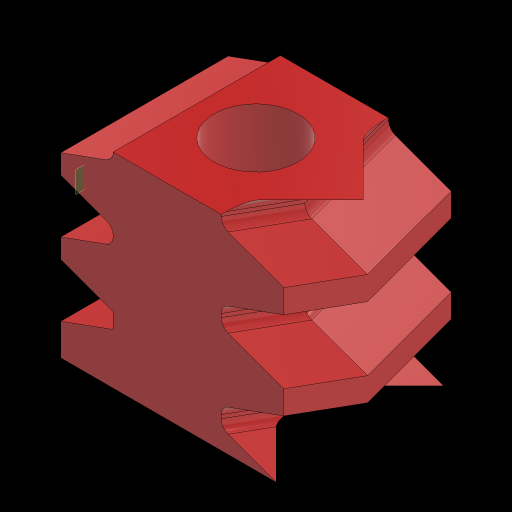
# Autodesk Inventor part: rack
Saved by Autodesk Inventor 2023.2 (Build 272271030, 271C)
## iProperties
Created: 2023-10-23
Part Number: rack
Material: Generic
Document SubType Name: Modeling
Designer: robpl
Density: 1 g/cm^3
Appearance: Red
Author: robpl
## iProperties of the stored document rack_3DPrint.ipt
Created: 2023-10-23
Part Number: rack_3DPrint
Material: Generic
Document SubType Name: Modeling
Designer: robpl
Density: 1 g/cm^3
Appearance: Default
Author: robpl
Autodesk Inventor part; units mm, degrees
ref_plane "YZ Plane" through (0, 0, 0) normal (1, 0, 0) x (0, 1, 0)
ref_plane "XZ Plane" through (0, 0, 0) normal (0, 1, 0) x (-1, 0, 0)
ref_plane "XY Plane" through (0, 0, 0) normal (0, 0, 1) x (1, 0, 0)
sketch "Sketch1" plane through (0, 0, 0) normal (0, 0, 1) x (1, 0, 0)
  line L0 (-6, -5.5) -> (6, -5.5)
  line L1 (6, -5.5) -> (6, 5.5)
  line L2 (6, 5.5) -> (-6, 5.5)
  line L3 (-6, 5.5) -> (-6, -5.5)
  point P0 (0, 0)
  point P1 (-6, 0)
  point P2 (0, 5.5)
  dimension "d0" = 12
  dimension "d1" = 11
  constraints: 8 end point, 2 midpoint, 2 parallel, 1 horizontal, 1 horizontal alignment, 1 perpendicular, 1 vertical alignment
  measures "d0" distance of L2.end L1.end
  measures "d1" distance of L1.end L0.end
extrude "Extrusion1" add sketch "Sketch1" along normal blind 4.5
sketch "Sketch2" plane through (0, 0, 4.5) normal (0, 0, 1) x (1, 0, 0)
  line L0 (6, -5.5) -> (6, 5.5) projected
  line L1 (6, 5.5) -> (-6, 5.5) projected
  line L2 (-6, 5.5) -> (-6, -5.5) projected
  line L3 (-6, -5.5) -> (6, -5.5) projected
  line L4 (6, -5.5) -> (6, 5.5) projected
  line L5 (6, 7.2241) -> (2.625, 5.9957)
  line L6 (2.625, 5.9957) -> (2.625, 5.0043)
  line L7 (2.625, 5.0043) -> (6, 3.7759)
  line L8 (6, 2.5117) -> (2.625, 1.2833)
  line L9 (2.625, 1.2833) -> (2.625, 0.292)
  line L10 (2.625, 0.292) -> (6, -0.9364)
  arc A0 (3, 6.1322) -> (2.625, 5.5965) centre (3.195, 5.5965) ccw
  arc A1 (2.625, 5.4035) -> (3, 4.8678) centre (3.195, 5.4035) ccw
  line L11 (6, 5.5) -> (-6, 5.5) projected
  arc A2 (2.625, 0.6911) -> (3, 0.1555) centre (3.195, 0.6911) ccw
  arc A3 (3, 1.4198) -> (2.625, 0.8841) centre (3.195, 0.8841) ccw
  line L12 (6, 7.2241) -> (6, 3.7759)
  line L13 (0, 5.5) -> (0.4792, -5.5)
  line L14 (0, -5.5) -> (6, -5.5) projected
  line L15 (-6.1272, 6.6958) -> (-2.6582, 5.7655)
  line L16 (-2.6582, 5.7655) -> (-2.572, 4.778)
  line L17 (-2.572, 4.778) -> (-5.8274, 3.2607)
  arc A4 (-2.6235, 5.3679) -> (-3.0437, 5.8689) centre (-3.1913, 5.3183) ccw
  arc A5 (-2.9337, 4.6094) -> (-2.6067, 5.1756) centre (-3.1745, 5.126) ccw
  line L18 (-6.1272, 6.6958) -> (-5.8274, 3.2607)
  line L19 (-5.7174, 2.0012) -> (-2.2484, 1.071)
  line L20 (-2.2484, 1.071) -> (-2.1622, 0.0834)
  line L21 (-2.1622, 0.0834) -> (-5.4176, -1.4338)
  arc A6 (-2.5239, -0.0852) -> (-2.1969, 0.481) centre (-2.7647, 0.4315) ccw
  arc A7 (-2.2137, 0.6734) -> (-2.6339, 1.1744) centre (-2.7815, 0.6238) ccw
  point P0 (0, 0)
  point P1 (0, 0)
  point P2 (2.625, 5.5)
  point P3 (4.5, 4.3219)
  point P4 (4.5, 1.9657)
  point P5 (2.625, 5.5)
  point P6 (6, -0.9364)
  point P7 (-2.6151, 5.2717)
  point P8 (-4.3805, 3.9351)
  point P9 (-6, 5.2386)
  point P10 (0, 7.2759)
  point P11 (-4.1756, 1.5878)
  point P12 (0, 2.5636)
  point P13 (0, 6.0117)
  point P14 (4.5, -0.3905)
  dimension "d14" = 70
  dimension "d15" = 4.7124
  dimension "d16" = 0.57
  dimension "d17" = 3.375
  dimension "d18" = 1.5
  dimension "d19" = 2.3562
  dimension "d48" = 2.3562
  constraints: 30 end point, 26 point on line, 23 symmetric about line, 16 point on circle, 8 centre point, 8 tangent, 4 equal length, 3 equal radius, 2 midpoint, 2 vertical, 2 vertical alignment, 1 parallel, 6 other
  measures "d14" angle of L0 L5
  measures "d15" distance of L10.end L7.end
  measures "d16" radius of A0
  measures "d17" distance between parallel lines of L6 L0
  measures "d18" distance from line of L0 point (4.5, 4.322)
  measures "d19" distance of point (4.5, 4.322) point (4.5, 1.966)
  measures "d48" distance of point (4.5, 1.966) point (4.5, -0.39)
sketch "Sketch3" plane through (6, -5.5, 0) normal (1, 0, 0) x (0, 0, -1)
  line L0 (-4.5, 0) -> (-4.5, 11) projected
  line L1 (-4.5, 11) -> (-4.5, 0) projected
  line L2 (-4.5, 4.5636) -> (0, 2.9257)
  line L3 (0, 5.5) -> (0, 11) projected
  line L4 (0, 11) -> (-4.5, 11) projected
  dimension "d31" = 20
  constraints: 2 end point, 1 point on line
  measures "d31" angle of L4 L2
sweep "Sweep1" cut profiles "Sketch2" path "Sketch3" path curves L2 contours L10 A2 L9 A3 L8 L0 | L7 A1 L6 L1 L0 | L6 A0 L5 L12 L1
pattern_linear "Rectangular Pattern2" count 8 spacing 4.7124 along (0, -1, 0) of "Sweep1"
mirror "Mirror2" about plane through (0, 0, 0) normal (0, 0, -1)
ref_plane "Work Plane3" through (4.5, 2.8745, 4.5) normal (1, 0, 0) x (0, 0, -1)
sketch "Sketch6" plane through (0, 0, 4.5) normal (0, 0, 1) x (1, 0, 0)
  arc A0 (3, -3.2926) -> (2.625, -3.8283) centre (3.195, -3.8283) ccw projected
  line L0 (3, -3.2926) -> (6, -2.2007) projected
  line L1 (6, -2.2007) -> (6, -0.9364) projected
  line L2 (6, -0.9364) -> (3, 0.1555) projected
  arc A1 (2.625, 0.6911) -> (3, 0.1555) centre (3.195, 0.6911) ccw projected
  line L3 (2.625, 0.6911) -> (2.625, 0.8841) projected
  arc A2 (3, 1.4198) -> (2.625, 0.8841) centre (3.195, 0.8841) ccw projected
  line L4 (3, 1.4198) -> (6, 2.5117) projected
  line L5 (6, 2.5117) -> (6, 3.7759) projected
  line L6 (6, 3.7759) -> (3, 4.8678) projected
  arc A3 (2.625, 5.4035) -> (3, 4.8678) centre (3.195, 5.4035) ccw projected
  line L7 (2.625, 5.4035) -> (2.625, 5.5) projected
  line L8 (2.625, 5.5) -> (-6, 5.5) projected
  line L9 (-6, 5.5) -> (-6, -5.5) projected
  line L10 (-6, -5.5) -> (5.5911, -5.5) projected
  line L11 (-6, 4.0633) -> (-3.1875, 5.087)
  line L12 (-3.1875, 5.087) -> (-3.1875, 5.913)
  line L13 (2.625, 5.5) -> (-6, 5.5) projected
  line L14 (-3.1875, 5.913) -> (-6, 6.9367)
  line L15 (-6, 6.9367) -> (-6, 5.5)
  arc A4 (-3.5, 4.9732) -> (-3.1875, 5.4196) centre (-3.6625, 5.4196) ccw
  arc A5 (-3.1875, 5.5804) -> (-3.5, 6.0268) centre (-3.6625, 5.5804) ccw
  arc A6 (-3.5, 1.0462) -> (-3.1875, 1.4926) centre (-3.6625, 1.4926) ccw
  line L16 (-3.1875, 1.16) -> (-3.1875, 1.9861)
  arc A7 (-3.1875, 1.6535) -> (-3.5, 2.0998) centre (-3.6625, 1.6535) ccw
  line L17 (-3.1875, 1.9861) -> (-6, 3.0097)
  line L18 (-6, 3.0097) -> (-6, 1.573)
  line L19 (-6, 0.1363) -> (-3.1875, 1.16)
  arc A8 (-3.5, -2.8808) -> (-3.1875, -2.4344) centre (-3.6625, -2.4344) ccw
  line L20 (-3.1875, -2.767) -> (-3.1875, -1.9409)
  arc A9 (-3.1875, -2.2735) -> (-3.5, -1.8272) centre (-3.6625, -2.2735) ccw
  line L21 (-3.1875, -1.9409) -> (-6, -0.9173)
  line L22 (-6, -0.9173) -> (-6, -2.354)
  line L23 (-6, -3.7907) -> (-3.1875, -2.767)
  arc A10 (-3.5, -6.8078) -> (-3.1875, -6.3614) centre (-3.6625, -6.3614) ccw
  line L24 (-3.1875, -6.694) -> (-3.1875, -5.8679)
  arc A11 (-3.1875, -6.2005) -> (-3.5, -5.7542) centre (-3.6625, -6.2005) ccw
  line L25 (-3.1875, -5.8679) -> (-6, -4.8443)
  line L26 (-6, -4.8443) -> (-6, -6.281)
  line L27 (-6, -7.7177) -> (-3.1875, -6.694)
  line L28 (5.5911, -5.5) -> (3, -4.5569) projected
  arc A12 (2.625, -4.0213) -> (3, -4.5569) centre (3.195, -4.0213) ccw projected
  line L29 (2.625, -4.0213) -> (2.625, -3.8283) projected
  point P0 (0, 0)
  point P1 (-4.75, 6.4817)
  point P2 (-4.75, 4.5183)
  point P3 (-3.1875, 5.5)
  point P4 (-3.1875, 1.573)
  point P5 (-4.75, 2.5548)
  point P6 (-4.75, 0.5913)
  point P7 (-3.1875, -2.354)
  point P8 (-4.75, -1.3722)
  point P9 (-4.75, -3.3357)
  point P10 (-3.1875, -6.281)
  point P11 (-4.75, -5.2992)
  point P12 (-4.75, -7.2627)
  point P13 (-5.2013, -4.5)
  dimension "d50" = 70
  dimension "d51" = 1.25
  dimension "d52" = 1.5625
  dimension "d53" = 1.9635
  dimension "d54" = 0.475
  dimension "d57" = 3.927
  constraints: 32 end point, 26 point on line, 16 point on circle, 8 centre point, 4 tangent, 1 equal length, 1 equal radius, 1 midpoint, 1 parallel, 1 perpendicular, 1 vertical, 1 vertical alignment, 60 other
  measures "d50" angle of L15 L14
  measures "d51" distance from line of L15 point (-4.75, 6.482)
  measures "d52" distance from line of point (-4.75, 6.482) L12
  measures "d53" distance of point (-4.75, 4.518) point (-4.75, 6.482)
  measures "d54" radius of A5
  measures "d57" distance of L11.end L16.start
extrude "Extrusion4" cut sketch "Sketch6" against normal blind 10 contours L9 L21 A9 L20 A8 L23 | A8 L20 L23 | L9 L17 A7 L16 A6 L19 | L21 L20 A9 | L12 A4 L11 L9 L8
ref_plane "Work Plane4" through (-4.75, 3.0097, -4.5) normal (-1, 0, 0) x (0, 0, 1)
sketch "Sketch7" plane through (0, 0, 0) normal (0, 1, 0) x (-1, 0, 0)
  circle A0 centre (0, 0) radius 2.25
  dimension "d65" = 4.5
  constraints: 2 coincident, 1 centre point
  measures "d65" diameter of A0
extrude "Extrusion5" cut sketch "Sketch7" along normal through all both and the other way through all
equation "\"d15\" = 3.14159 * d18"
equation "\"d16\" = 0.38 * d18"
equation "\"d17\" = 2.25 * d18"
equation "\"d19\" = 0.5 * d15"
equation "\"d48\" = d19"
equation "\"d52\" = 1.25 * d51"
equation "\"d53\" = 1.5708 * d51"
equation "\"d54\" = 0.38 * d51"
equation "\"d57\" = 3.14159 * d51"
equation "\"d32\" = 20.5deg"
body "Solid1"
